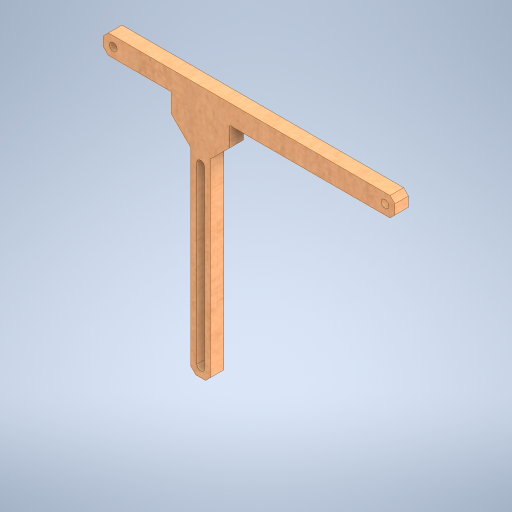
# Autodesk Inventor part: tLever
Saved by Autodesk Inventor 2023.1 (Build 271208000, 208)
## iProperties
Created: 2022-10-28
Part Number: tLever
Material: MDF Medium Density Fiberboard
Document SubType Name: Modeling
Designer: Daniel Peña
Density: 0.8 g/cm^3
Appearance: Cherry - Natural Low Gloss
Author: Daniel Peña
Autodesk Inventor part; units mm, degrees
ref_plane "YZ Plane" through (0, 0, 0) normal (1, 0, 0) x (0, 1, 0)
ref_plane "XZ Plane" through (0, 0, 0) normal (0, 1, 0) x (-1, 0, 0)
ref_plane "XY Plane" through (0, 0, 0) normal (0, 0, 1) x (1, 0, 0)
sketch "Sketch1" plane through (0, 0, 0) normal (0, 0, 1) x (1, 0, 0)
  line L0 (-11.8764, 47.9805) -> (133.1236, 47.9805) projected
  line L1 (133.1236, 47.9805) -> (135.6236, 50.4805) projected
  line L2 (135.6236, 50.4805) -> (135.6236, 55.4805) projected
  line L3 (135.6236, 55.4805) -> (133.1236, 57.9805) projected
  line L4 (133.1236, 57.9805) -> (75.6236, 57.9805) projected
  line L5 (-11.8764, 57.9805) -> (-14.3764, 55.4805) projected
  line L6 (-14.3764, 55.4805) -> (-14.3764, 50.4805) projected
  line L7 (-14.3764, 50.4805) -> (-11.8764, 47.9805) projected
  line L8 (75.6236, 57.9805) -> (75.6236, 67.9805) projected
  line L9 (75.6236, 67.9805) -> (65.6236, 77.9805) projected
  line L10 (65.6236, 77.9805) -> (55.6236, 77.9805) projected
  line L11 (55.6236, 77.9805) -> (45.6236, 67.9805) projected
  line L12 (45.6236, 67.9805) -> (45.6236, 57.9805) projected
  line L13 (45.6236, 57.9805) -> (-11.8764, 57.9805) projected
  circle A0 centre (-9.3764, 52.9805) radius 2 projected
  circle A1 centre (130.6236, 52.9805) radius 2 projected
  line L14 (200.7921, 30.8795) -> (340.7921, 30.8795) construction
  line L15 (245.7921, 30.8795) -> (245.7921, -89.1205) construction
  line L16 (198.2921, 35.8795) -> (343.2921, 35.8795)
  line L17 (240.7921, 5.8795) -> (240.7921, -91.6205)
  line L18 (250.7921, 5.8795) -> (250.7921, -91.6205)
  line L19 (248.2921, -94.1205) -> (243.2921, -94.1205)
  line L20 (195.7921, 33.3795) -> (195.7921, 28.3795)
  line L21 (345.7921, 33.3795) -> (345.7921, 28.3795)
  line L22 (240.7921, -91.6205) -> (243.2921, -94.1205)
  line L23 (250.7921, -91.6205) -> (248.2921, -94.1205)
  line L24 (343.2921, 25.8795) -> (345.7921, 28.3795)
  line L25 (345.7921, 33.3795) -> (343.2921, 35.8795)
  line L26 (198.2921, 35.8795) -> (195.7921, 33.3795)
  line L27 (195.7921, 28.3795) -> (198.2921, 25.8795)
  line L28 (198.2921, 25.8795) -> (230.7921, 25.8795)
  line L29 (260.7921, 25.8795) -> (343.2921, 25.8795)
  line L30 (260.7921, 25.8795) -> (260.7921, 15.8795)
  line L31 (230.7921, 15.8795) -> (230.7921, 25.8795)
  line L32 (250.7921, 5.8795) -> (260.7921, 15.8795)
  line L33 (240.7921, 5.8795) -> (230.7921, 15.8795)
  point P0 (195.7921, 35.8795)
  point P1 (345.7921, 35.8795)
  point P2 (195.7921, 25.8795)
  point P3 (345.7921, 25.8795)
  point P4 (240.7921, -94.1205)
  point P5 (250.7921, -94.1205)
  point P6 (260.7921, 5.8795)
  point P7 (230.7921, 5.8795)
  dimension "d54" = 140
  dimension "d55" = 120
  dimension "d56" = 45
  dimension "d57" = 5
  dimension "d59" = 5
  dimension "d60" = 5
  dimension "d61" = 5
  dimension "d62" = 5
  dimension "d63" = 5
  dimension "d64" = 2.5
  dimension "d65" = 2.5
  dimension "d66" = 2.5
  dimension "d67" = 2.5
  dimension "d68" = 2.5
  dimension "d69" = 2.5
  dimension "d70" = 2.5
  dimension "d71" = 2.5
  dimension "d72" = 2.5
  dimension "d73" = 2.5
  dimension "d74" = 2.5
  dimension "d75" = 2.5
  dimension "d76" = 30
  dimension "d77" = 20
  dimension "d78" = 15
  dimension "d79" = 10
  dimension "d80" = 10
  dimension "d81" = 10
  dimension "d82" = 10
  constraints: 40 end point, 13 point on line, 6 parallel, 3 vertical, 2 horizontal
  measures "d54" distance of L14.start L14.end
  measures "d55" distance of L15.start L15.end
  measures "d56" distance from line of L14.start L15
  measures "d57" distance between parallel lines of L14 L16
  measures "d59" distance between parallel lines of L15 L17
  measures "d60" distance between parallel lines of L15 L18
  measures "d61" distance from line of L15.end L19
  measures "d62" distance from line of L20 L14.start
  measures "d63" distance from line of L14.end L21
  measures "d64" distance of L17.end point (240.792, -94.12)
  measures "d65" distance of L19.end point (240.792, -94.12)
  measures "d66" distance of L18.end point (250.792, -94.12)
  measures "d67" distance of L19.start point (250.792, -94.12)
  measures "d68" distance of L24.start point (345.792, 25.88)
  measures "d69" distance of L21.end point (345.792, 25.88)
  measures "d70" distance of L21.start point (345.792, 35.88)
  measures "d71" distance of L16.end point (345.792, 35.88)
  measures "d72" distance of L16.start point (195.792, 35.88)
  measures "d73" distance of L20.start point (195.792, 35.88)
  measures "d74" distance of L20.end point (195.792, 25.88)
  measures "d75" distance of L27.end point (195.792, 25.88)
  measures "d76" distance of point (260.792, 5.88) point (230.792, 5.88)
  measures "d77" distance of L29.start point (260.792, 5.88)
  measures "d78" distance between parallel lines of L15 L30
  measures "d79" distance of L18.start point (260.792, 5.88)
  measures "d80" distance of L30.end point (260.792, 5.88)
  measures "d81" distance of L17.start point (230.792, 5.88)
  measures "d82" distance of L31.start point (230.792, 5.88)
extrude "Extrusion1" add sketch "Sketch1" along normal blind 7 contours L16 L25 L21 L24 L29 L30 L32 L18 L23 L19 L22 L17 L33 L31 L28 L27 L20 L26
sketch "Sketch2" plane through (0, 0, 7) normal (0, 0, 1) x (1, 0, 0)
  line L0 (195.7921, 33.3795) -> (195.7921, 28.3795) projected
  line L1 (345.7921, 28.3795) -> (345.7921, 33.3795) projected
  point P0 (200.7921, 30.8795)
  point P1 (340.7921, 30.8795)
  dimension "d83" = 5
  dimension "d84" = 5
  measures "d83" distance from line of L0 point (200.792, 30.88)
  measures "d84" distance from line of L1 point (340.792, 30.88)
hole "Hole1" at (200.7921, 30.8795, 7) at (340.7921, 30.8795, 7) direction (0, 0, -1) diameter 4 end through all
sketch "Sketch4" plane through (0, 0, 7) normal (0, 0, 1) x (1, 0, 0)
  circle A0 centre (200.7921, 30.8795) radius 2 construction
  circle A1 centre (340.7921, 30.8795) radius 2 construction
  line L0 (200.7921, 30.8795) -> (340.7921, 30.8795) construction
  line L1 (245.7921, -89.1205) -> (245.7921, 30.8795) construction
  line L2 (243.2921, -94.1205) -> (248.2921, -94.1205) construction
  line L3 (243.7921, -89.1205) -> (243.7921, 0.8795)
  line L4 (247.7921, 0.8795) -> (247.7921, -89.1205)
  arc A2 (247.7921, 0.8795) -> (243.7921, 0.8795) centre (245.7921, 0.8795) ccw
  arc A3 (243.7921, -89.1205) -> (247.7921, -89.1205) centre (245.7921, -89.1205) ccw
  point P0 (0, 0)
  point P1 (245.7921, -94.1205)
  dimension "d89" = 2
  dimension "d90" = 45
  dimension "d92" = 5
  dimension "d93" = 2
  constraints: 8 end point, 4 point on circle, 4 tangent, 2 centre point, 1 equal radius, 1 horizontal, 1 midpoint, 1 parallel, 1 perpendicular, 1 point on line
  measures "d89" radius of A2
  measures "d90" distance from line of L0.start L1
  measures "d92" distance of point (245.792, -94.12) L1.start
  measures "d93" distance between parallel lines of L4 L1
extrude "Extrusion3" cut sketch "Sketch4" against normal blind 7
equation "\"d65\" = d64"
equation "\"d66\" = d64"
equation "\"d67\" = d66"
equation "\"d68\" = d64"
equation "\"d69\" = d68"
equation "\"d70\" = d64"
equation "\"d71\" = d70"
equation "\"d72\" = d64"
equation "\"d73\" = d72"
equation "\"d74\" = d64"
equation "\"d75\" = d74"
equation "\"d80\" = d79"
equation "\"d81\" = d79"
equation "\"d82\" = d81"
body "Solid1"
